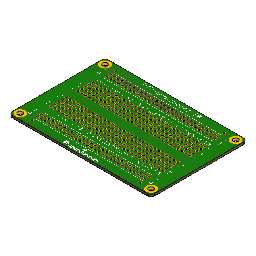
Battery Welder Box v6 (Autodesk Fusion 360 archive; units mm, degrees)
design "SIK-DIP-board"
part number: STANDOFF_ELECTRICAL
part number: LOGO-SFECP
part number: LOGO-SFENEW
part number: M29NO_SILK
part number: OSHW-LOGOS
part number: M01SMDNS
Autodesk Fusion 360 part; units mm, degrees
sketch "sketch 305" plane through (0, 0, 0) normal (0, 0, 1) x (1, 0, 0)
  line L0 (0, 61.178) -> (0, 2.322)
  arc A0 (0, 2.322) -> (2.322, 0) centre (2.322, 2.322) ccw
  line L1 (2.322, 0) -> (91.658, 0)
  arc A1 (91.658, 0) -> (93.98, 2.322) centre (91.658, 2.322) ccw
  line L2 (93.98, 2.322) -> (93.98, 61.178)
  arc A2 (93.98, 61.178) -> (91.658, 63.5) centre (91.658, 61.178) ccw
  line L3 (91.658, 63.5) -> (2.322, 63.5)
  arc A3 (2.322, 63.5) -> (0, 61.178) centre (2.322, 61.178) ccw
extrude "Board" add sketch "sketch 305" along normal blind 1.57 makes body 1 in component "Board"
sketch "sketch 3117" plane through (0, 0, 0) normal (0, 0, 1) x (1, 0, 0)
  line L0 (-1.6, -1.6) -> (1.6, -1.6)
  line L1 (1.6, -1.6) -> (1.6, 1.6)
  line L2 (1.6, 1.6) -> (-1.6, 1.6)
  line L3 (-1.6, 1.6) -> (-1.6, -1.6)
extrude "STANDOFF-ELECTRICAL" add sketch "sketch 3117" along normal blind 0.1 separate body makes body 2 in component "STANDOFF-ELECTRICAL"
sketch "sketch 3721" plane through (0, 0, 0) normal (0, 0, 1) x (1, 0, 0)
  line L0 (-0.508, -0.508) -> (10.668, -0.508)
  line L1 (10.668, -0.508) -> (10.668, 0.508)
  line L2 (10.668, 0.508) -> (-0.508, 0.508)
  line L3 (-0.508, 0.508) -> (-0.508, -0.508)
extrude "1X05_NO_SILK" add sketch "sketch 3721" along normal blind 0.1 separate body makes body 3 in component "1X05_NO_SILK"
sketch "sketch 3853" plane through (0, 0, 0) normal (0, 0, 1) x (1, 0, 0)
  line L0 (0, 0.002) -> (1.859, 0.002)
  line L1 (1.859, 0.002) -> (1.859, 2.804)
  line L2 (1.859, 2.804) -> (0, 2.804)
  line L3 (0, 2.804) -> (0, 0.002)
extrude "SFE-LOGO-FLAME-COPPER" add sketch "sketch 3853" along normal blind 0.1 separate body makes body 4 in component "SFE-LOGO-FLAME-COPPER"
sketch "sketch 3985" plane through (0, 0, 0) normal (0, 0, 1) x (1, 0, 0)
  line L0 (0.013, 0.018) -> (19.037, 0.018)
  line L1 (19.037, 0.018) -> (19.037, 5.687)
  line L2 (19.037, 5.687) -> (0.013, 5.687)
  line L3 (0.013, 5.687) -> (0.013, 0.018)
extrude "SFE-NEW-WEBLOGO" add sketch "sketch 3985" along normal blind 0.1 separate body makes body 5 in component "SFE-NEW-WEBLOGO"
sketch "sketch 4141" plane through (0, 0, 0) normal (0, 0, 1) x (1, 0, 0)
  line L0 (-0.508, -0.508) -> (71.628, -0.508)
  line L1 (71.628, -0.508) -> (71.628, 0.508)
  line L2 (71.628, 0.508) -> (-0.508, 0.508)
  line L3 (-0.508, 0.508) -> (-0.508, -0.508)
extrude "1X29_NO_SILK" add sketch "sketch 4141" along normal blind 0.1 separate body makes body 6 in component "1X29_NO_SILK"
sketch "sketch 4273" plane through (0, 0, 0) normal (0, 0, 1) x (1, 0, 0)
  line L0 (-1.489, -1.182) -> (1.489, -1.182)
  line L1 (1.489, -1.182) -> (1.489, 1.489)
  line L2 (1.489, 1.489) -> (-1.489, 1.489)
  line L3 (-1.489, 1.489) -> (-1.489, -1.182)
extrude "OSHW-LOGO-S" add sketch "sketch 4273" along normal blind 0.1 separate body makes body 7 in component "OSHW-LOGO-S"
sketch "sketch 4429" plane through (0, 0, 0) normal (0, 0, 1) x (1, 0, 0)
  line L0 (-0.508, -0.508) -> (0.508, -0.508)
  line L1 (0.508, -0.508) -> (0.508, 0.508)
  line L2 (0.508, 0.508) -> (-0.508, 0.508)
  line L3 (-0.508, 0.508) -> (-0.508, -0.508)
extrude "1X01NS" add sketch "sketch 4429" along normal blind 0.1 separate body makes body 8 in component "1X01NS"
sketch "sketch 437" plane through (0, 0, 0) normal (0, 0, 1) x (1, 0, 0)
  circle A0 centre (3.81, 59.69) radius 1.6
  circle A1 centre (90.17, 59.69) radius 1.6
  circle A2 centre (3.81, 3.81) radius 1.6
  circle A3 centre (90.17, 3.81) radius 1.6
  circle A4 centre (22.86, 17.78) radius 0.508
  circle A5 centre (22.86, 20.32) radius 0.508
  circle A6 centre (22.86, 22.86) radius 0.508
  circle A7 centre (22.86, 25.4) radius 0.508
  circle A8 centre (22.86, 27.94) radius 0.508
  circle A9 centre (10.16, 17.78) radius 0.508
  circle A10 centre (10.16, 20.32) radius 0.508
  circle A11 centre (10.16, 22.86) radius 0.508
  circle A12 centre (10.16, 25.4) radius 0.508
  circle A13 centre (10.16, 27.94) radius 0.508
  circle A14 centre (12.7, 17.78) radius 0.508
  circle A15 centre (12.7, 20.32) radius 0.508
  circle A16 centre (12.7, 22.86) radius 0.508
  circle A17 centre (12.7, 25.4) radius 0.508
  circle A18 centre (12.7, 27.94) radius 0.508
  circle A19 centre (15.24, 17.78) radius 0.508
  circle A20 centre (15.24, 20.32) radius 0.508
  circle A21 centre (15.24, 22.86) radius 0.508
  circle A22 centre (15.24, 25.4) radius 0.508
  circle A23 centre (15.24, 27.94) radius 0.508
  circle A24 centre (17.78, 17.78) radius 0.508
  circle A25 centre (17.78, 20.32) radius 0.508
  circle A26 centre (17.78, 22.86) radius 0.508
  circle A27 centre (17.78, 25.4) radius 0.508
  circle A28 centre (17.78, 27.94) radius 0.508
  circle A29 centre (20.32, 17.78) radius 0.508
  circle A30 centre (20.32, 20.32) radius 0.508
  circle A31 centre (20.32, 22.86) radius 0.508
  circle A32 centre (20.32, 25.4) radius 0.508
  circle A33 centre (20.32, 27.94) radius 0.508
  circle A34 centre (25.4, 17.78) radius 0.508
  circle A35 centre (25.4, 20.32) radius 0.508
  circle A36 centre (25.4, 22.86) radius 0.508
  circle A37 centre (25.4, 25.4) radius 0.508
  circle A38 centre (25.4, 27.94) radius 0.508
  circle A39 centre (27.94, 17.78) radius 0.508
  circle A40 centre (27.94, 20.32) radius 0.508
  circle A41 centre (27.94, 22.86) radius 0.508
  circle A42 centre (27.94, 25.4) radius 0.508
  circle A43 centre (27.94, 27.94) radius 0.508
  circle A44 centre (30.48, 17.78) radius 0.508
  circle A45 centre (30.48, 20.32) radius 0.508
  circle A46 centre (30.48, 22.86) radius 0.508
  circle A47 centre (30.48, 25.4) radius 0.508
  circle A48 centre (30.48, 27.94) radius 0.508
  circle A49 centre (33.02, 17.78) radius 0.508
  circle A50 centre (33.02, 20.32) radius 0.508
  circle A51 centre (33.02, 22.86) radius 0.508
  circle A52 centre (33.02, 25.4) radius 0.508
  circle A53 centre (33.02, 27.94) radius 0.508
  circle A54 centre (35.56, 17.78) radius 0.508
  circle A55 centre (35.56, 20.32) radius 0.508
  circle A56 centre (35.56, 22.86) radius 0.508
  circle A57 centre (35.56, 25.4) radius 0.508
  circle A58 centre (35.56, 27.94) radius 0.508
  circle A59 centre (38.1, 17.78) radius 0.508
  circle A60 centre (38.1, 20.32) radius 0.508
  circle A61 centre (38.1, 22.86) radius 0.508
  circle A62 centre (38.1, 25.4) radius 0.508
  circle A63 centre (38.1, 27.94) radius 0.508
  circle A64 centre (40.64, 17.78) radius 0.508
  circle A65 centre (40.64, 20.32) radius 0.508
  circle A66 centre (40.64, 22.86) radius 0.508
  circle A67 centre (40.64, 25.4) radius 0.508
  circle A68 centre (40.64, 27.94) radius 0.508
  circle A69 centre (43.18, 17.78) radius 0.508
  circle A70 centre (43.18, 20.32) radius 0.508
  circle A71 centre (43.18, 22.86) radius 0.508
  circle A72 centre (43.18, 25.4) radius 0.508
  circle A73 centre (43.18, 27.94) radius 0.508
  circle A74 centre (45.72, 17.78) radius 0.508
  circle A75 centre (45.72, 20.32) radius 0.508
  circle A76 centre (45.72, 22.86) radius 0.508
  circle A77 centre (45.72, 25.4) radius 0.508
  circle A78 centre (45.72, 27.94) radius 0.508
  circle A79 centre (48.26, 17.78) radius 0.508
  circle A80 centre (48.26, 20.32) radius 0.508
  circle A81 centre (48.26, 22.86) radius 0.508
  circle A82 centre (48.26, 25.4) radius 0.508
  circle A83 centre (48.26, 27.94) radius 0.508
  circle A84 centre (50.8, 17.78) radius 0.508
  circle A85 centre (50.8, 20.32) radius 0.508
  circle A86 centre (50.8, 22.86) radius 0.508
  circle A87 centre (50.8, 25.4) radius 0.508
  circle A88 centre (50.8, 27.94) radius 0.508
  circle A89 centre (53.34, 17.78) radius 0.508
  circle A90 centre (53.34, 20.32) radius 0.508
  circle A91 centre (53.34, 22.86) radius 0.508
  circle A92 centre (53.34, 25.4) radius 0.508
  circle A93 centre (53.34, 27.94) radius 0.508
  circle A94 centre (55.88, 17.78) radius 0.508
  circle A95 centre (55.88, 20.32) radius 0.508
  circle A96 centre (55.88, 22.86) radius 0.508
  circle A97 centre (55.88, 25.4) radius 0.508
  circle A98 centre (55.88, 27.94) radius 0.508
  circle A99 centre (58.42, 17.78) radius 0.508
  circle A100 centre (58.42, 20.32) radius 0.508
  circle A101 centre (58.42, 22.86) radius 0.508
  circle A102 centre (58.42, 25.4) radius 0.508
  circle A103 centre (58.42, 27.94) radius 0.508
  circle A104 centre (60.96, 17.78) radius 0.508
  circle A105 centre (60.96, 20.32) radius 0.508
  circle A106 centre (60.96, 22.86) radius 0.508
  circle A107 centre (60.96, 25.4) radius 0.508
  circle A108 centre (60.96, 27.94) radius 0.508
  circle A109 centre (63.5, 17.78) radius 0.508
  circle A110 centre (63.5, 20.32) radius 0.508
  circle A111 centre (63.5, 22.86) radius 0.508
  circle A112 centre (63.5, 25.4) radius 0.508
  circle A113 centre (63.5, 27.94) radius 0.508
  circle A114 centre (66.04, 17.78) radius 0.508
  circle A115 centre (66.04, 20.32) radius 0.508
  circle A116 centre (66.04, 22.86) radius 0.508
  circle A117 centre (66.04, 25.4) radius 0.508
  circle A118 centre (66.04, 27.94) radius 0.508
  circle A119 centre (68.58, 17.78) radius 0.508
  circle A120 centre (68.58, 20.32) radius 0.508
  circle A121 centre (68.58, 22.86) radius 0.508
  circle A122 centre (68.58, 25.4) radius 0.508
  circle A123 centre (68.58, 27.94) radius 0.508
  circle A124 centre (71.12, 17.78) radius 0.508
  circle A125 centre (71.12, 20.32) radius 0.508
  circle A126 centre (71.12, 22.86) radius 0.508
  circle A127 centre (71.12, 25.4) radius 0.508
  circle A128 centre (71.12, 27.94) radius 0.508
  circle A129 centre (73.66, 17.78) radius 0.508
  circle A130 centre (73.66, 20.32) radius 0.508
  circle A131 centre (73.66, 22.86) radius 0.508
  circle A132 centre (73.66, 25.4) radius 0.508
  circle A133 centre (73.66, 27.94) radius 0.508
  circle A134 centre (76.2, 17.78) radius 0.508
  circle A135 centre (76.2, 20.32) radius 0.508
  circle A136 centre (76.2, 22.86) radius 0.508
  circle A137 centre (76.2, 25.4) radius 0.508
  circle A138 centre (76.2, 27.94) radius 0.508
  circle A139 centre (78.74, 17.78) radius 0.508
  circle A140 centre (78.74, 20.32) radius 0.508
  circle A141 centre (78.74, 22.86) radius 0.508
  circle A142 centre (78.74, 25.4) radius 0.508
  circle A143 centre (78.74, 27.94) radius 0.508
  circle A144 centre (81.28, 17.78) radius 0.508
  circle A145 centre (81.28, 20.32) radius 0.508
  circle A146 centre (81.28, 22.86) radius 0.508
  circle A147 centre (81.28, 25.4) radius 0.508
  circle A148 centre (81.28, 27.94) radius 0.508
  circle A149 centre (83.82, 17.78) radius 0.508
  circle A150 centre (83.82, 20.32) radius 0.508
  circle A151 centre (83.82, 22.86) radius 0.508
  circle A152 centre (83.82, 25.4) radius 0.508
  circle A153 centre (83.82, 27.94) radius 0.508
  circle A154 centre (10.16, 35.56) radius 0.508
  circle A155 centre (10.16, 38.1) radius 0.508
  circle A156 centre (10.16, 40.64) radius 0.508
  circle A157 centre (10.16, 43.18) radius 0.508
  circle A158 centre (10.16, 45.72) radius 0.508
  circle A159 centre (12.7, 35.56) radius 0.508
  circle A160 centre (12.7, 38.1) radius 0.508
  circle A161 centre (12.7, 40.64) radius 0.508
  circle A162 centre (12.7, 43.18) radius 0.508
  circle A163 centre (12.7, 45.72) radius 0.508
  circle A164 centre (15.24, 35.56) radius 0.508
  circle A165 centre (15.24, 38.1) radius 0.508
  circle A166 centre (15.24, 40.64) radius 0.508
  circle A167 centre (15.24, 43.18) radius 0.508
  circle A168 centre (15.24, 45.72) radius 0.508
  circle A169 centre (17.78, 35.56) radius 0.508
  circle A170 centre (17.78, 38.1) radius 0.508
  circle A171 centre (17.78, 40.64) radius 0.508
  circle A172 centre (17.78, 43.18) radius 0.508
  circle A173 centre (17.78, 45.72) radius 0.508
  circle A174 centre (20.32, 35.56) radius 0.508
  circle A175 centre (20.32, 38.1) radius 0.508
  circle A176 centre (20.32, 40.64) radius 0.508
  circle A177 centre (20.32, 43.18) radius 0.508
  circle A178 centre (20.32, 45.72) radius 0.508
  circle A179 centre (22.86, 35.56) radius 0.508
  circle A180 centre (22.86, 38.1) radius 0.508
  circle A181 centre (22.86, 40.64) radius 0.508
  circle A182 centre (22.86, 43.18) radius 0.508
  circle A183 centre (22.86, 45.72) radius 0.508
  circle A184 centre (25.4, 35.56) radius 0.508
  circle A185 centre (25.4, 38.1) radius 0.508
  circle A186 centre (25.4, 40.64) radius 0.508
  circle A187 centre (25.4, 43.18) radius 0.508
  circle A188 centre (25.4, 45.72) radius 0.508
  circle A189 centre (27.94, 35.56) radius 0.508
  circle A190 centre (27.94, 38.1) radius 0.508
  circle A191 centre (27.94, 40.64) radius 0.508
  circle A192 centre (27.94, 43.18) radius 0.508
  circle A193 centre (27.94, 45.72) radius 0.508
  circle A194 centre (30.48, 35.56) radius 0.508
  circle A195 centre (30.48, 38.1) radius 0.508
  circle A196 centre (30.48, 40.64) radius 0.508
  circle A197 centre (30.48, 43.18) radius 0.508
  circle A198 centre (30.48, 45.72) radius 0.508
  circle A199 centre (33.02, 35.56) radius 0.508
  circle A200 centre (33.02, 38.1) radius 0.508
  circle A201 centre (33.02, 40.64) radius 0.508
  circle A202 centre (33.02, 43.18) radius 0.508
  circle A203 centre (33.02, 45.72) radius 0.508
  circle A204 centre (35.56, 35.56) radius 0.508
  circle A205 centre (35.56, 38.1) radius 0.508
  circle A206 centre (35.56, 40.64) radius 0.508
  circle A207 centre (35.56, 43.18) radius 0.508
  circle A208 centre (35.56, 45.72) radius 0.508
  circle A209 centre (40.64, 35.56) radius 0.508
  circle A210 centre (40.64, 38.1) radius 0.508
  circle A211 centre (40.64, 40.64) radius 0.508
  circle A212 centre (40.64, 43.18) radius 0.508
  circle A213 centre (40.64, 45.72) radius 0.508
  circle A214 centre (38.1, 35.56) radius 0.508
  circle A215 centre (38.1, 38.1) radius 0.508
  circle A216 centre (38.1, 40.64) radius 0.508
  circle A217 centre (38.1, 43.18) radius 0.508
  circle A218 centre (38.1, 45.72) radius 0.508
  circle A219 centre (43.18, 35.56) radius 0.508
  circle A220 centre (43.18, 38.1) radius 0.508
  circle A221 centre (43.18, 40.64) radius 0.508
  circle A222 centre (43.18, 43.18) radius 0.508
  circle A223 centre (43.18, 45.72) radius 0.508
  circle A224 centre (45.72, 35.56) radius 0.508
  circle A225 centre (45.72, 38.1) radius 0.508
  circle A226 centre (45.72, 40.64) radius 0.508
  circle A227 centre (45.72, 43.18) radius 0.508
  circle A228 centre (45.72, 45.72) radius 0.508
  circle A229 centre (48.26, 35.56) radius 0.508
  circle A230 centre (48.26, 38.1) radius 0.508
  circle A231 centre (48.26, 40.64) radius 0.508
  circle A232 centre (48.26, 43.18) radius 0.508
  circle A233 centre (48.26, 45.72) radius 0.508
  circle A234 centre (50.8, 35.56) radius 0.508
  circle A235 centre (50.8, 38.1) radius 0.508
  circle A236 centre (50.8, 40.64) radius 0.508
  circle A237 centre (50.8, 43.18) radius 0.508
  circle A238 centre (50.8, 45.72) radius 0.508
  circle A239 centre (53.34, 35.56) radius 0.508
  circle A240 centre (53.34, 38.1) radius 0.508
  circle A241 centre (53.34, 40.64) radius 0.508
  circle A242 centre (53.34, 43.18) radius 0.508
  circle A243 centre (53.34, 45.72) radius 0.508
  circle A244 centre (55.88, 35.56) radius 0.508
  circle A245 centre (55.88, 38.1) radius 0.508
  circle A246 centre (55.88, 40.64) radius 0.508
  circle A247 centre (55.88, 43.18) radius 0.508
  circle A248 centre (55.88, 45.72) radius 0.508
  circle A249 centre (58.42, 35.56) radius 0.508
  circle A250 centre (58.42, 38.1) radius 0.508
  circle A251 centre (58.42, 40.64) radius 0.508
  circle A252 centre (58.42, 43.18) radius 0.508
  circle A253 centre (58.42, 45.72) radius 0.508
  circle A254 centre (60.96, 35.56) radius 0.508
  circle A255 centre (60.96, 38.1) radius 0.508
  circle A256 centre (60.96, 40.64) radius 0.508
  circle A257 centre (60.96, 43.18) radius 0.508
  circle A258 centre (60.96, 45.72) radius 0.508
  circle A259 centre (63.5, 35.56) radius 0.508
  circle A260 centre (63.5, 38.1) radius 0.508
  circle A261 centre (63.5, 40.64) radius 0.508
  circle A262 centre (63.5, 43.18) radius 0.508
  circle A263 centre (63.5, 45.72) radius 0.508
  circle A264 centre (66.04, 35.56) radius 0.508
  circle A265 centre (66.04, 38.1) radius 0.508
  circle A266 centre (66.04, 40.64) radius 0.508
  circle A267 centre (66.04, 43.18) radius 0.508
  circle A268 centre (66.04, 45.72) radius 0.508
  circle A269 centre (68.58, 35.56) radius 0.508
  circle A270 centre (68.58, 38.1) radius 0.508
  circle A271 centre (68.58, 40.64) radius 0.508
  circle A272 centre (68.58, 43.18) radius 0.508
  circle A273 centre (68.58, 45.72) radius 0.508
  circle A274 centre (71.12, 35.56) radius 0.508
  circle A275 centre (71.12, 38.1) radius 0.508
  circle A276 centre (71.12, 40.64) radius 0.508
  circle A277 centre (71.12, 43.18) radius 0.508
  circle A278 centre (71.12, 45.72) radius 0.508
  circle A279 centre (73.66, 35.56) radius 0.508
  circle A280 centre (73.66, 38.1) radius 0.508
  circle A281 centre (73.66, 40.64) radius 0.508
  circle A282 centre (73.66, 43.18) radius 0.508
  circle A283 centre (73.66, 45.72) radius 0.508
  circle A284 centre (76.2, 35.56) radius 0.508
  circle A285 centre (76.2, 38.1) radius 0.508
  circle A286 centre (76.2, 40.64) radius 0.508
  circle A287 centre (76.2, 43.18) radius 0.508
  circle A288 centre (76.2, 45.72) radius 0.508
  circle A289 centre (78.74, 35.56) radius 0.508
  circle A290 centre (78.74, 38.1) radius 0.508
  circle A291 centre (78.74, 40.64) radius 0.508
  circle A292 centre (78.74, 43.18) radius 0.508
  circle A293 centre (78.74, 45.72) radius 0.508
  circle A294 centre (81.28, 35.56) radius 0.508
  circle A295 centre (81.28, 38.1) radius 0.508
  circle A296 centre (81.28, 40.64) radius 0.508
  circle A297 centre (81.28, 43.18) radius 0.508
  circle A298 centre (81.28, 45.72) radius 0.508
  circle A299 centre (83.82, 35.56) radius 0.508
  circle A300 centre (83.82, 38.1) radius 0.508
  circle A301 centre (83.82, 40.64) radius 0.508
  circle A302 centre (83.82, 43.18) radius 0.508
  circle A303 centre (83.82, 45.72) radius 0.508
  circle A304 centre (11.43, 55.88) radius 0.508
  circle A305 centre (13.97, 55.88) radius 0.508
  circle A306 centre (16.51, 55.88) radius 0.508
  circle A307 centre (19.05, 55.88) radius 0.508
  circle A308 centre (21.59, 55.88) radius 0.508
  circle A309 centre (24.13, 55.88) radius 0.508
  circle A310 centre (26.67, 55.88) radius 0.508
  circle A311 centre (29.21, 55.88) radius 0.508
  circle A312 centre (31.75, 55.88) radius 0.508
  circle A313 centre (34.29, 55.88) radius 0.508
  circle A314 centre (36.83, 55.88) radius 0.508
  circle A315 centre (39.37, 55.88) radius 0.508
  circle A316 centre (41.91, 55.88) radius 0.508
  circle A317 centre (44.45, 55.88) radius 0.508
  circle A318 centre (46.99, 55.88) radius 0.508
  circle A319 centre (49.53, 55.88) radius 0.508
  circle A320 centre (52.07, 55.88) radius 0.508
  circle A321 centre (54.61, 55.88) radius 0.508
  circle A322 centre (57.15, 55.88) radius 0.508
  circle A323 centre (59.69, 55.88) radius 0.508
  circle A324 centre (62.23, 55.88) radius 0.508
  circle A325 centre (64.77, 55.88) radius 0.508
  circle A326 centre (67.31, 55.88) radius 0.508
  circle A327 centre (69.85, 55.88) radius 0.508
  circle A328 centre (72.39, 55.88) radius 0.508
  circle A329 centre (74.93, 55.88) radius 0.508
  circle A330 centre (77.47, 55.88) radius 0.508
  circle A331 centre (80.01, 55.88) radius 0.508
  circle A332 centre (82.55, 55.88) radius 0.508
  circle A333 centre (11.43, 53.34) radius 0.508
  circle A334 centre (13.97, 53.34) radius 0.508
  circle A335 centre (16.51, 53.34) radius 0.508
  circle A336 centre (19.05, 53.34) radius 0.508
  circle A337 centre (21.59, 53.34) radius 0.508
  circle A338 centre (24.13, 53.34) radius 0.508
  circle A339 centre (26.67, 53.34) radius 0.508
  circle A340 centre (29.21, 53.34) radius 0.508
  circle A341 centre (31.75, 53.34) radius 0.508
  circle A342 centre (34.29, 53.34) radius 0.508
  circle A343 centre (36.83, 53.34) radius 0.508
  circle A344 centre (39.37, 53.34) radius 0.508
  circle A345 centre (41.91, 53.34) radius 0.508
  circle A346 centre (44.45, 53.34) radius 0.508
  circle A347 centre (46.99, 53.34) radius 0.508
  circle A348 centre (49.53, 53.34) radius 0.508
  circle A349 centre (52.07, 53.34) radius 0.508
  circle A350 centre (54.61, 53.34) radius 0.508
  circle A351 centre (57.15, 53.34) radius 0.508
  circle A352 centre (59.69, 53.34) radius 0.508
  circle A353 centre (62.23, 53.34) radius 0.508
  circle A354 centre (64.77, 53.34) radius 0.508
  circle A355 centre (67.31, 53.34) radius 0.508
  circle A356 centre (69.85, 53.34) radius 0.508
  circle A357 centre (72.39, 53.34) radius 0.508
  circle A358 centre (74.93, 53.34) radius 0.508
  circle A359 centre (77.47, 53.34) radius 0.508
  circle A360 centre (80.01, 53.34) radius 0.508
  circle A361 centre (82.55, 53.34) radius 0.508
  circle A362 centre (11.43, 10.16) radius 0.508
  circle A363 centre (13.97, 10.16) radius 0.508
  circle A364 centre (16.51, 10.16) radius 0.508
  circle A365 centre (19.05, 10.16) radius 0.508
  circle A366 centre (21.59, 10.16) radius 0.508
  circle A367 centre (24.13, 10.16) radius 0.508
  circle A368 centre (26.67, 10.16) radius 0.508
  circle A369 centre (29.21, 10.16) radius 0.508
  circle A370 centre (31.75, 10.16) radius 0.508
  circle A371 centre (34.29, 10.16) radius 0.508
  circle A372 centre (36.83, 10.16) radius 0.508
  circle A373 centre (39.37, 10.16) radius 0.508
  circle A374 centre (41.91, 10.16) radius 0.508
  circle A375 centre (44.45, 10.16) radius 0.508
  circle A376 centre (46.99, 10.16) radius 0.508
  circle A377 centre (49.53, 10.16) radius 0.508
  circle A378 centre (52.07, 10.16) radius 0.508
  circle A379 centre (54.61, 10.16) radius 0.508
  circle A380 centre (57.15, 10.16) radius 0.508
  circle A381 centre (59.69, 10.16) radius 0.508
  circle A382 centre (62.23, 10.16) radius 0.508
  circle A383 centre (64.77, 10.16) radius 0.508
  circle A384 centre (67.31, 10.16) radius 0.508
  circle A385 centre (69.85, 10.16) radius 0.508
  circle A386 centre (72.39, 10.16) radius 0.508
  circle A387 centre (74.93, 10.16) radius 0.508
  circle A388 centre (77.47, 10.16) radius 0.508
  circle A389 centre (80.01, 10.16) radius 0.508
  circle A390 centre (82.55, 10.16) radius 0.508
  circle A391 centre (11.43, 7.62) radius 0.508
  circle A392 centre (13.97, 7.62) radius 0.508
  circle A393 centre (16.51, 7.62) radius 0.508
  circle A394 centre (19.05, 7.62) radius 0.508
  circle A395 centre (21.59, 7.62) radius 0.508
  circle A396 centre (24.13, 7.62) radius 0.508
  circle A397 centre (26.67, 7.62) radius 0.508
  circle A398 centre (29.21, 7.62) radius 0.508
  circle A399 centre (31.75, 7.62) radius 0.508
  circle A400 centre (34.29, 7.62) radius 0.508
  circle A401 centre (36.83, 7.62) radius 0.508
  circle A402 centre (39.37, 7.62) radius 0.508
  circle A403 centre (41.91, 7.62) radius 0.508
  circle A404 centre (44.45, 7.62) radius 0.508
  circle A405 centre (46.99, 7.62) radius 0.508
  circle A406 centre (49.53, 7.62) radius 0.508
  circle A407 centre (52.07, 7.62) radius 0.508
  circle A408 centre (54.61, 7.62) radius 0.508
  circle A409 centre (57.15, 7.62) radius 0.508
  circle A410 centre (59.69, 7.62) radius 0.508
  circle A411 centre (62.23, 7.62) radius 0.508
  circle A412 centre (64.77, 7.62) radius 0.508
  circle A413 centre (67.31, 7.62) radius 0.508
  circle A414 centre (69.85, 7.62) radius 0.508
  circle A415 centre (72.39, 7.62) radius 0.508
  circle A416 centre (74.93, 7.62) radius 0.508
  circle A417 centre (77.47, 7.62) radius 0.508
  circle A418 centre (80.01, 7.62) radius 0.508
  circle A419 centre (82.55, 7.62) radius 0.508
  circle A420 centre (82.55, 59.69) radius 0.508
  circle A421 centre (11.43, 59.69) radius 0.508
  circle A422 centre (11.43, 3.81) radius 0.508
  circle A423 centre (82.55, 3.81) radius 0.508
extrude "Extrude2" cut sketch "sketch 437" along normal blind 1.57 bodies 1 in component "Board"
component "PCB Component" placed x (1, 0, 0) y (0, 1, 0) z (0, 0, 1) at (0, 0, 0)
component "Board" placed x (1, 0, 0) y (0, 1, 0) z (0, 0, 1) at (0, 0, 0) in component "PCB Component"
component "STANDOFF-ELECTRICAL" placed x (1, 0, 0) y (0, 1, 0) z (0, 0, 1) at (3.81, 59.69, 1.57) in component "PCB Component"
component "STANDOFF-ELECTRICAL" placed x (1, 0, 0) y (0, 1, 0) z (0, 0, 1) at (90.17, 59.69, 1.57) in component "PCB Component"
component "STANDOFF-ELECTRICAL" placed x (1, 0, 0) y (0, 1, 0) z (0, 0, 1) at (3.81, 3.81, 1.57) in component "PCB Component"
component "STANDOFF-ELECTRICAL" placed x (1, 0, 0) y (0, 1, 0) z (0, 0, 1) at (90.17, 3.81, 1.57) in component "PCB Component"
component "1X05_NO_SILK" placed x (0, 1, 0) y (-1, 0, 0) z (0, 0, 1) at (22.86, 17.78, 1.57) in component "PCB Component"
component "1X05_NO_SILK" placed x (0, 1, 0) y (-1, 0, 0) z (0, 0, 1) at (10.16, 17.78, 1.57) in component "PCB Component"
component "1X05_NO_SILK" placed x (0, 1, 0) y (-1, 0, 0) z (0, 0, 1) at (12.7, 17.78, 1.57) in component "PCB Component"
component "1X05_NO_SILK" placed x (0, 1, 0) y (-1, 0, 0) z (0, 0, 1) at (15.24, 17.78, 1.57) in component "PCB Component"
component "1X05_NO_SILK" placed x (0, 1, 0) y (-1, 0, 0) z (0, 0, 1) at (17.78, 17.78, 1.57) in component "PCB Component"
component "1X05_NO_SILK" placed x (0, 1, 0) y (-1, 0, 0) z (0, 0, 1) at (20.32, 17.78, 1.57) in component "PCB Component"
component "1X05_NO_SILK" placed x (0, 1, 0) y (-1, 0, 0) z (0, 0, 1) at (25.4, 17.78, 1.57) in component "PCB Component"
component "1X05_NO_SILK" placed x (0, 1, 0) y (-1, 0, 0) z (0, 0, 1) at (27.94, 17.78, 1.57) in component "PCB Component"
component "1X05_NO_SILK" placed x (0, 1, 0) y (-1, 0, 0) z (0, 0, 1) at (30.48, 17.78, 1.57) in component "PCB Component"
component "1X05_NO_SILK" placed x (0, 1, 0) y (-1, 0, 0) z (0, 0, 1) at (33.02, 17.78, 1.57) in component "PCB Component"
component "1X05_NO_SILK" placed x (0, 1, 0) y (-1, 0, 0) z (0, 0, 1) at (35.56, 17.78, 1.57) in component "PCB Component"
component "1X05_NO_SILK" placed x (0, 1, 0) y (-1, 0, 0) z (0, 0, 1) at (38.1, 17.78, 1.57) in component "PCB Component"
component "1X05_NO_SILK" placed x (0, 1, 0) y (-1, 0, 0) z (0, 0, 1) at (40.64, 17.78, 1.57) in component "PCB Component"
component "1X05_NO_SILK" placed x (0, 1, 0) y (-1, 0, 0) z (0, 0, 1) at (43.18, 17.78, 1.57) in component "PCB Component"
component "1X05_NO_SILK" placed x (0, 1, 0) y (-1, 0, 0) z (0, 0, 1) at (45.72, 17.78, 1.57) in component "PCB Component"
component "1X05_NO_SILK" placed x (0, 1, 0) y (-1, 0, 0) z (0, 0, 1) at (48.26, 17.78, 1.57) in component "PCB Component"
component "1X05_NO_SILK" placed x (0, 1, 0) y (-1, 0, 0) z (0, 0, 1) at (50.8, 17.78, 1.57) in component "PCB Component"
component "1X05_NO_SILK" placed x (0, 1, 0) y (-1, 0, 0) z (0, 0, 1) at (53.34, 17.78, 1.57) in component "PCB Component"
component "1X05_NO_SILK" placed x (0, 1, 0) y (-1, 0, 0) z (0, 0, 1) at (55.88, 17.78, 1.57) in component "PCB Component"
component "1X05_NO_SILK" placed x (0, 1, 0) y (-1, 0, 0) z (0, 0, 1) at (58.42, 17.78, 1.57) in component "PCB Component"
component "1X05_NO_SILK" placed x (0, 1, 0) y (-1, 0, 0) z (0, 0, 1) at (60.96, 17.78, 1.57) in component "PCB Component"
component "1X05_NO_SILK" placed x (0, 1, 0) y (-1, 0, 0) z (0, 0, 1) at (63.5, 17.78, 1.57) in component "PCB Component"
component "1X05_NO_SILK" placed x (0, 1, 0) y (-1, 0, 0) z (0, 0, 1) at (66.04, 17.78, 1.57) in component "PCB Component"
component "1X05_NO_SILK" placed x (0, 1, 0) y (-1, 0, 0) z (0, 0, 1) at (68.58, 17.78, 1.57) in component "PCB Component"
component "1X05_NO_SILK" placed x (0, 1, 0) y (-1, 0, 0) z (0, 0, 1) at (71.12, 17.78, 1.57) in component "PCB Component"
component "1X05_NO_SILK" placed x (0, 1, 0) y (-1, 0, 0) z (0, 0, 1) at (73.66, 17.78, 1.57) in component "PCB Component"
component "1X05_NO_SILK" placed x (0, 1, 0) y (-1, 0, 0) z (0, 0, 1) at (76.2, 17.78, 1.57) in component "PCB Component"
component "1X05_NO_SILK" placed x (0, 1, 0) y (-1, 0, 0) z (0, 0, 1) at (78.74, 17.78, 1.57) in component "PCB Component"
component "1X05_NO_SILK" placed x (0, 1, 0) y (-1, 0, 0) z (0, 0, 1) at (81.28, 17.78, 1.57) in component "PCB Component"
component "1X05_NO_SILK" placed x (0, 1, 0) y (-1, 0, 0) z (0, 0, 1) at (83.82, 17.78, 1.57) in component "PCB Component"
component "1X05_NO_SILK" placed x (0, 1, 0) y (-1, 0, 0) z (0, 0, 1) at (10.16, 35.56, 1.57) in component "PCB Component"
component "1X05_NO_SILK" placed x (0, 1, 0) y (-1, 0, 0) z (0, 0, 1) at (12.7, 35.56, 1.57) in component "PCB Component"
component "1X05_NO_SILK" placed x (0, 1, 0) y (-1, 0, 0) z (0, 0, 1) at (15.24, 35.56, 1.57) in component "PCB Component"
component "1X05_NO_SILK" placed x (0, 1, 0) y (-1, 0, 0) z (0, 0, 1) at (17.78, 35.56, 1.57) in component "PCB Component"
component "1X05_NO_SILK" placed x (0, 1, 0) y (-1, 0, 0) z (0, 0, 1) at (20.32, 35.56, 1.57) in component "PCB Component"
component "1X05_NO_SILK" placed x (0, 1, 0) y (-1, 0, 0) z (0, 0, 1) at (22.86, 35.56, 1.57) in component "PCB Component"
component "1X05_NO_SILK" placed x (0, 1, 0) y (-1, 0, 0) z (0, 0, 1) at (25.4, 35.56, 1.57) in component "PCB Component"
component "1X05_NO_SILK" placed x (0, 1, 0) y (-1, 0, 0) z (0, 0, 1) at (27.94, 35.56, 1.57) in component "PCB Component"
component "1X05_NO_SILK" placed x (0, 1, 0) y (-1, 0, 0) z (0, 0, 1) at (30.48, 35.56, 1.57) in component "PCB Component"
component "1X05_NO_SILK" placed x (0, 1, 0) y (-1, 0, 0) z (0, 0, 1) at (33.02, 35.56, 1.57) in component "PCB Component"
component "1X05_NO_SILK" placed x (0, 1, 0) y (-1, 0, 0) z (0, 0, 1) at (35.56, 35.56, 1.57) in component "PCB Component"
component "1X05_NO_SILK" placed x (0, 1, 0) y (-1, 0, 0) z (0, 0, 1) at (40.64, 35.56, 1.57) in component "PCB Component"
component "1X05_NO_SILK" placed x (0, 1, 0) y (-1, 0, 0) z (0, 0, 1) at (38.1, 35.56, 1.57) in component "PCB Component"
component "1X05_NO_SILK" placed x (0, 1, 0) y (-1, 0, 0) z (0, 0, 1) at (43.18, 35.56, 1.57) in component "PCB Component"
component "1X05_NO_SILK" placed x (0, 1, 0) y (-1, 0, 0) z (0, 0, 1) at (45.72, 35.56, 1.57) in component "PCB Component"
component "1X05_NO_SILK" placed x (0, 1, 0) y (-1, 0, 0) z (0, 0, 1) at (48.26, 35.56, 1.57) in component "PCB Component"
component "1X05_NO_SILK" placed x (0, 1, 0) y (-1, 0, 0) z (0, 0, 1) at (50.8, 35.56, 1.57) in component "PCB Component"
component "1X05_NO_SILK" placed x (0, 1, 0) y (-1, 0, 0) z (0, 0, 1) at (53.34, 35.56, 1.57) in component "PCB Component"
component "1X05_NO_SILK" placed x (0, 1, 0) y (-1, 0, 0) z (0, 0, 1) at (55.88, 35.56, 1.57) in component "PCB Component"
component "1X05_NO_SILK" placed x (0, 1, 0) y (-1, 0, 0) z (0, 0, 1) at (58.42, 35.56, 1.57) in component "PCB Component"
component "1X05_NO_SILK" placed x (0, 1, 0) y (-1, 0, 0) z (0, 0, 1) at (60.96, 35.56, 1.57) in component "PCB Component"
component "1X05_NO_SILK" placed x (0, 1, 0) y (-1, 0, 0) z (0, 0, 1) at (63.5, 35.56, 1.57) in component "PCB Component"
component "1X05_NO_SILK" placed x (0, 1, 0) y (-1, 0, 0) z (0, 0, 1) at (66.04, 35.56, 1.57) in component "PCB Component"
component "1X05_NO_SILK" placed x (0, 1, 0) y (-1, 0, 0) z (0, 0, 1) at (68.58, 35.56, 1.57) in component "PCB Component"
component "1X05_NO_SILK" placed x (0, 1, 0) y (-1, 0, 0) z (0, 0, 1) at (71.12, 35.56, 1.57) in component "PCB Component"
component "1X05_NO_SILK" placed x (0, 1, 0) y (-1, 0, 0) z (0, 0, 1) at (73.66, 35.56, 1.57) in component "PCB Component"
component "1X05_NO_SILK" placed x (0, 1, 0) y (-1, 0, 0) z (0, 0, 1) at (76.2, 35.56, 1.57) in component "PCB Component"
component "1X05_NO_SILK" placed x (0, 1, 0) y (-1, 0, 0) z (0, 0, 1) at (78.74, 35.56, 1.57) in component "PCB Component"
component "1X05_NO_SILK" placed x (0, 1, 0) y (-1, 0, 0) z (0, 0, 1) at (81.28, 35.56, 1.57) in component "PCB Component"
component "1X05_NO_SILK" placed x (0, 1, 0) y (-1, 0, 0) z (0, 0, 1) at (83.82, 35.56, 1.57) in component "PCB Component"
component "SFE-LOGO-FLAME-COPPER" placed x (-1, 0, 0) y (0, 1, 0) z (0, 0, -1) at (46.99, 1.27, 0) in component "PCB Component"
component "SFE-NEW-WEBLOGO" placed x (1, 0, 0) y (0, 1, 0) z (0, 0, 1) at (38.1, 0, 1.57) in component "PCB Component"
component "1X29_NO_SILK" placed x (1, 0, 0) y (0, 1, 0) z (0, 0, 1) at (11.43, 55.88, 1.57) in component "PCB Component"
component "1X29_NO_SILK" placed x (1, 0, 0) y (0, 1, 0) z (0, 0, 1) at (11.43, 53.34, 1.57) in component "PCB Component"
component "1X29_NO_SILK" placed x (1, 0, 0) y (0, 1, 0) z (0, 0, 1) at (11.43, 10.16, 1.57) in component "PCB Component"
component "1X29_NO_SILK" placed x (1, 0, 0) y (0, 1, 0) z (0, 0, 1) at (11.43, 7.62, 1.57) in component "PCB Component"
component "OSHW-LOGO-S" placed x (1, 0, 0) y (0, 1, 0) z (0, 0, 1) at (35.56, 2.54, 1.57) in component "PCB Component"
component "1X01NS" placed x (1, 0, 0) y (0, 1, 0) z (0, 0, 1) at (82.55, 59.69, 1.57) in component "PCB Component"
component "1X01NS" placed x (1, 0, 0) y (0, 1, 0) z (0, 0, 1) at (11.43, 59.69, 1.57) in component "PCB Component"
component "1X01NS" placed x (1, 0, 0) y (0, 1, 0) z (0, 0, 1) at (11.43, 3.81, 1.57) in component "PCB Component"
component "1X01NS" placed x (1, 0, 0) y (0, 1, 0) z (0, 0, 1) at (82.55, 3.81, 1.57) in component "PCB Component"
hidden bodies 2 4 7 8
named bodies: "Board", "STANDOFF-ELECTRICAL", "1X05_NO_SILK", "SFE-LOGO-FLAME-COPPER", "SFE-NEW-WEBLOGO", "1X29_NO_SILK", "OSHW-LOGO-S", "1X01NS"
